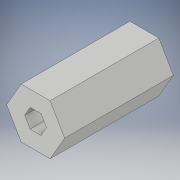
# Autodesk Inventor part: HexSpacer
Saved by Autodesk Inventor 2019 (Build 230136000, 136)
## iProperties
Created: 2019-02-09
Part Number: HexSpacer
Material: Generic
Document SubType Name: Modeling
Designer: james
Density: 1 g/cm^3
Appearance: Default
Author: james
Autodesk Inventor part; units mm, degrees
ref_plane "YZ Plane" through (0, 0, 0) normal (1, 0, 0) x (0, 1, 0)
ref_plane "XZ Plane" through (0, 0, 0) normal (0, 1, 0) x (-1, 0, 0)
ref_plane "XY Plane" through (0, 0, 0) normal (0, 0, 1) x (1, 0, 0)
sketch "Sketch2" plane through (0, 0, 0) normal (0, 0, 1) x (1, 0, 0)
  line L0 (7.62, 0) -> (3.81, -6.5991)
  line L1 (3.81, -6.5991) -> (-3.81, -6.5991)
  line L2 (-3.81, -6.5991) -> (-7.62, 0)
  line L3 (-7.62, 0) -> (-3.81, 6.5991)
  line L4 (-3.81, 6.5991) -> (3.81, 6.5991)
  line L5 (3.81, 6.5991) -> (7.62, 0)
  line L6 (20.32, 0) -> (10.16, -17.5976)
  line L7 (10.16, -17.5976) -> (-10.16, -17.5976)
  line L8 (-10.16, -17.5976) -> (-20.32, 0)
  line L9 (-20.32, 0) -> (-10.16, 17.5976)
  line L10 (-10.16, 17.5976) -> (10.16, 17.5976)
  line L11 (10.16, 17.5976) -> (20.32, 0)
  point P0 (0, 0)
  point P1 (0, 0)
  point P2 (0, 0)
  dimension "d2" = 7.62
  dimension "d3" = 20.32
  constraints: 24 end point, 2 coincident, 26 other
  measures "d2" distance of L3.end L4.end
  measures "d3" distance of L9.end L10.end
extrude "Extrusion1" add sketch "Sketch2" along normal blind 76.2
body "Solid1"
